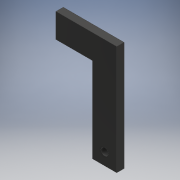
# Autodesk Inventor part: makerbeam_L-bracket
Saved by Autodesk Inventor 2018 (Build 220112000, 112)
## iProperties
Created: 2017-11-16
Part Number: makerbeam_L-bracket
Material: Acetal Resin, Black
Document SubType Name: Modeling
Designer: g
Density: 1.425 g/cm^3
Appearance: Smooth - Black
Author: g
Autodesk Inventor part; units mm, degrees
ref_plane "YZ Plane" through (0, 0, 0) normal (1, 0, 0) x (0, 1, 0)
ref_plane "XZ Plane" through (0, 0, 0) normal (0, 1, 0) x (-1, 0, 0)
ref_plane "XY Plane" through (0, 0, 0) normal (0, 0, 1) x (1, 0, 0)
sketch "Sketch1" plane through (0, 0, 0) normal (0, 1, 0) x (-1, 0, 0)
  line L0 (0, 0) -> (10, 0)
  line L1 (10, -10) -> (10, -45)
  line L2 (10, -45) -> (0, -45)
  line L3 (0, -45) -> (0, 0)
  line L4 (0, 0) -> (25, 0)
  line L5 (25, 0) -> (25, -10)
  line L6 (25, -10) -> (10, -10)
  line L7 (0, -10) -> (0, 0)
  dimension "d0" = 10
  dimension "d1" = 45
  dimension "d3" = 10
  dimension "d6" = 25
  constraints: 16 end point, 4 parallel, 2 horizontal, 2 perpendicular
  measures "d0" distance of L1.end L2.end
  measures "d1" distance of L0.end L1.end
  measures "d3" distance of L4.end L5.end
  measures "d6" distance between parallel lines of L3 L5
extrude "Extrusion1" add sketch "Sketch1" along normal blind 3
sketch "Sketch2" plane through (0, 3, 0) normal (0, 1, 0) x (1, 0, 0)
  line L0 (0, 45) -> (-10, 45) construction
  line L1 (-10, 45) -> (0, 35) construction
  line L2 (0, 0) -> (0, 45) construction
  line L3 (0, 45) -> (-10, 35) construction
  line L4 (-10, 45) -> (-10, 10) construction
  circle A0 centre (-5, 40) radius 1.5
  dimension "d7" = 135
  dimension "d8" = 45
  dimension "d9" = 3
  constraints: 4 end point, 2 point on line, 1 centre point, 1 midpoint
  measures "d7" angle of L0 L3
  measures "d8" angle of L0 L1
  measures "d9" diameter of A0
extrude "Extrusion2" cut sketch "Sketch2" against normal blind 10
body "Solid1"
